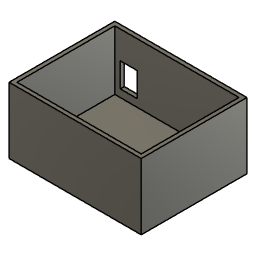
container v2 (Autodesk Fusion 360 archive; units mm, degrees)
design "cont"
Autodesk Fusion 360 part; units mm, degrees
sketch "Sketch1" plane through (0, 0, 0) normal (0, 1, 0) x (1, 0, 0)
  line L0 (50, -40) -> (-50, -40)
  line L1 (-50, -40) -> (-50, 40)
  line L2 (-50, 40) -> (50, 40)
  line L3 (50, 40) -> (50, -40)
  line L4 (50, -40) -> (-50, 40) construction
  line L5 (-50, -40) -> (50, 40) construction
  dimension "d1" = 100
  dimension "d2" = 80
  constraint horizontal L0
  constraint perpendicular L0 L1
  constraint parallel L0 L2
  constraint parallel L1 L3
  constraint coincident L4 origin
  constraint coincident L5 origin
  measures "d1" distance of L1.end L2.end
  measures "d2" distance of L0.end L1.end
extrude "Extrude1" add sketch "Sketch1" along normal blind 50
sketch "Sketch2" plane through (0, 50, 0) normal (0, 1, 0) x (-1, 0, 0)
  line L0 (-50, -40) -> (50, -40)
  line L1 (50, -40) -> (50, 40)
  line L2 (50, 40) -> (-50, 40)
  line L3 (-50, 40) -> (-50, -40)
  line L4 (-47, 37) -> (47, 37)
  line L5 (47, 37) -> (47, -37)
  line L6 (47, -37) -> (-47, -37)
  line L7 (-47, -37) -> (-47, 37)
  line L8 (-47, 37) -> (47, -37) construction
  line L9 (47, 37) -> (-47, -37) construction
  dimension "d5" = 94
  dimension "d6" = 74
  dimension "d15" = 3
  dimension "d16" = 3
  constraint horizontal L4
  constraint perpendicular L4 L5
  constraint parallel L4 L6
  constraint parallel L5 L7
  constraint coincident L8 origin
  constraint coincident L9 origin
  measures "d5" distance of L5.end L6.end
  measures "d6" distance of L4.end L5.end
  measures "d15" distance of L0 L6
  measures "d16" distance of L1 L5
extrude "Extrude4" cut sketch "Sketch2" against normal blind 45 contours L4 L5 L6 L7
sketch "Sketch5" plane through (0, 0, -37) normal (0, 0, 1) x (1, 0, 0)
  line L0 (47, 50) -> (-47, 50)
  line L1 (-47, 50) -> (-47, 5)
  line L2 (-47, 5) -> (47, 5)
  line L3 (47, 5) -> (47, 50)
  line L4 (-42.8809, 29.1227) -> (-30.0809, 29.1227)
  line L5 (-30.0809, 29.1227) -> (-30.0809, 10.7227)
  line L6 (-30.0809, 10.7227) -> (-42.8809, 10.7227)
  line L7 (-42.8809, 10.7227) -> (-42.8809, 29.1227)
  dimension "d19" = 12.8
  dimension "d20" = 18.4
  constraint horizontal L4
  constraint vertical L5
  constraint horizontal L6
  constraint vertical L7
  measures "d19" distance of L4.start L4.end
  measures "d20" distance of L4.start L6.end
extrude "Extrude5" cut sketch "Sketch5" against normal blind 55 contours L4 L5 L6 L7
extrude "Extrude2" [rolled back] along distance -45 taper angle 0
sketch "Sketch3" plane through (0, 0, -40) normal (0, 0, -1) x (-1, 0, 0)
  line L0 (-50, 0) -> (50, 0)
  line L1 (50, 0) -> (50, 50)
  line L2 (50, 50) -> (-50, 50)
  line L3 (-50, 50) -> (-50, 0)
  line L4 (-45, 5) -> (-32.2, 5)
  line L5 (-32.2, 5) -> (-32.2, 23.4)
  line L6 (-32.2, 23.4) -> (-45, 23.4)
  line L7 (-45, 23.4) -> (-45, 5)
  dimension "d11" = 12.8
  dimension "d12" = 18.4
  constraint horizontal L4
  constraint vertical L5
  constraint horizontal L6
  constraint vertical L7
  measures "d11" distance of L4.start L4.end
  measures "d12" distance of L4.start L6.end
extrude "Extrude3" [rolled back] along distance -10 taper angle 0
